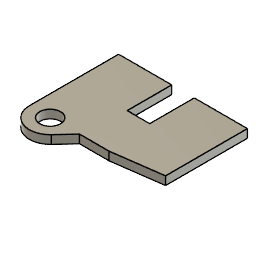
constraints (Autodesk Fusion 360 design; units mm, degrees)
Autodesk Fusion 360 part; units mm, degrees
sketch "Constraints Demo" plane through (0, 0, 0) normal (0, 1, 0) x (1, 0, 0)
  line L0 (41.0664, 18.1324) -> (104.0349, 18.1324)
  line L1 (104.0349, 18.1324) -> (104.0349, -34.6359)
  line L2 (104.0349, -34.6359) -> (130.6094, -34.6359)
  line L3 (130.6094, -34.6359) -> (130.6094, 18.1324)
  line L4 (130.6094, 18.1324) -> (193.5779, 18.1324)
  line L5 (193.5779, 18.1324) -> (193.5779, -78.8329)
  line L6 (193.5779, -78.8329) -> (134.7794, -86.972)
  line L7 (134.7794, -86.972) -> (99.8649, -86.972)
  line L8 (99.8649, -86.972) -> (83.789, -104.2824)
  line L9 (41.0664, 18.1324) -> (41.0664, -87.5042)
  arc A0 (41.0664, -87.5042) -> (83.789, -104.2824) centre (65.7223, -87.5042) ccw
  circle A1 centre (65.7223, -87.5042) radius 12.3567
  line L10 (117.3222, -86.972) -> (117.3222, -34.6359)
  line L11 (250, -100) -> (250, -35)
  spline S0 degree 5 poles (250, -35) (250, -32.6028) (250, -27.8084) (250.0776, -20.8345) (250.5826, -12.5726) (252.2639, -4.5288) (255.2107, 1.2852) (259.5207, 5.2526) (265.2004, 7.8511) (272.1693, 9.4403) (280.3152, 10.2655) (287.6902, 10.4323) (293.6726, 10.3106) (297.858, 10.1215) (300, 10) knots 0 0 0 0 0 0 0.1 0.2 0.3 0.4 0.5 0.6 0.7 0.8 0.9 1 1 1 1 1 1
  point P0 (260, 5)
  constraint vertical L10
  constraint horizontal L0
  constraint horizontal L4
  constraint coincident L2 L10.end
  constraint tangent L9 A0
  constraint tangent L8 A0
  constraint equal L0 L4
  constraint parallel L3 L5
  constraint perpendicular L4 L9
  constraint perpendicular L0 L1
  constraint perpendicular L1 L2
  constraint midpoint L7 L10.start
  constraint midpoint L2 L10.end
  constraint perpendicular L7 L10
  constraint concentric A0 A1
  constraint collinear L0 L4
  constraint vertical L11
extrude "Extrude1" add sketch "Constraints Demo" along normal blind 10
